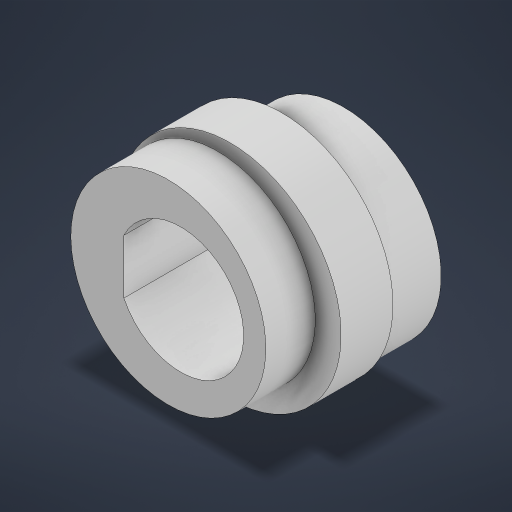
# Autodesk Inventor part: EccentricBearingShaft
Saved by Autodesk Inventor 2024 (Build 280153000, 153)
## iProperties
Created: 2024-01-30
Part Number: EccentricBearingShaft
Material: Generic
Document SubType Name: Modeling
Designer: avsar
Density: 1 g/cm^3
Appearance: Default
Author: avsar
Autodesk Inventor part; units mm, degrees
ref_plane "YZ Plane" through (0, 0, 0) normal (1, 0, 0) x (0, 1, 0)
ref_plane "XZ Plane" through (0, 0, 0) normal (0, 1, 0) x (-1, 0, 0)
ref_plane "XY Plane" through (0, 0, 0) normal (0, 0, 1) x (1, 0, 0)
sketch "Sketch1" plane through (0, 0, 0) normal (0, 0, 1) x (1, 0, 0)
  arc A0 (-4.5, -2.1795) -> (-4.5, 2.1795) centre (0, 0) ccw construction
  line L0 (-4.5, 2.1795) -> (-4.5, -2.1795) construction
  arc A1 (-4.5, 2.1795) -> (-4.5, -2.1795) centre (0, 0) ccw construction
  arc A2 (-4.6, -2.2023) -> (-4.6, 2.2023) centre (0, 0) ccw
  line L1 (-4.6, -2.2023) -> (-4.6, 2.2023)
  circle A3 centre (0, 0) radius 8
  dimension "d0" = 10
  dimension "d1" = 4.359
  dimension "d2" = 0.1
  dimension "d3" = 16
  constraints: 6 point on circle, 4 centre point, 4 end point, 2 coincident, 1 vertical, 1 other
  measures "d0" diameter of A0
  measures "d1" distance of L0.start L0.end
  measures "d2" radial gap between concentric circles of A0 A2
  measures "d3" diameter of A3
extrude "Extrusion1" add sketch "Sketch1" along normal blind 4
sketch "Sketch2" plane through (0, 0, 0) normal (0, 0, -1) x (-1, 0, 0)
  circle A0 centre (1, 0) radius 7.9
  arc A1 (4.6, 2.2023) -> (4.6, -2.2023) centre (0, 0) ccw projected
  line L0 (4.6, -2.2023) -> (4.6, 2.2023) projected
  dimension "d6" = 15.8
  dimension "d7" = 1
  constraints: 1 centre point, 1 horizontal alignment
  measures "d6" diameter of A0
  measures "d7" distance of A0.centre point (0, 0)
extrude "Extrusion2" add sketch "Sketch2" along normal blind 4
sketch "Sketch5" plane through (0, 0, 4) normal (0, 0, 1) x (1, 0, 0)
  circle A0 centre (0, 0) radius 8 projected
extrude "Extrusion5" cut sketch "Sketch5" against normal up to surface (4 mm away)
sketch "Sketch6" plane through (-1, 0, -4) normal (0, 0, -1) x (-1, 0, 0)
  circle A0 centre (-1, 0) radius 9
  arc A1 (3.6, 2.2023) -> (3.6, -2.2023) centre (-1, 0) ccw projected
  line L0 (3.6, 2.2023) -> (3.6, -2.2023) projected
  dimension "d19" = 18
  constraints: 1 centre point, 1 coincident
  measures "d19" diameter of A0
extrude "Extrusion6" add sketch "Sketch6" along normal blind 4.2
sketch "Sketch7" plane through (0, 0, -8.2) normal (0, 0, -1) x (-1, 0, 0)
  circle A0 centre (-1, 0) radius 7.9
  arc A1 (4.6, 2.2023) -> (4.6, -2.2023) centre (0, 0) ccw projected
  line L0 (4.6, 2.2023) -> (4.6, -2.2023) projected
  dimension "d22" = 15.8
  dimension "d23" = 1
  constraints: 1 centre point, 1 horizontal alignment
  measures "d22" diameter of A0
  measures "d23" distance of point (0, 0) A0.centre
extrude "Extrusion7" add sketch "Sketch7" along normal blind 4
body "Solid1"
